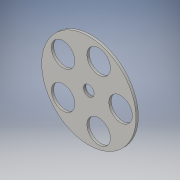
# Autodesk Inventor part: Drehplatte_Rahmenvorrrichtung
Saved by Autodesk Inventor 2016 (Build 200138000, 138)
## iProperties
Created: 2017-09-29
Part Number: Drehplatte_Rahmenvorrrichtung
Material: Generisch
Document SubType Name: Modeling
Designer: Dominik
Density: 1 g/cm^3
Appearance: Vorgabe
Author: Dominik
Autodesk Inventor part; units mm, degrees
ref_plane "YZ Plane" through (0, 0, 0) normal (1, 0, 0) x (0, 1, 0)
ref_plane "XZ Plane" through (0, 0, 0) normal (0, 1, 0) x (-1, 0, 0)
ref_plane "XY Plane" through (0, 0, 0) normal (0, 0, 1) x (1, 0, 0)
sketch "Skizze1" plane through (0, 0, 0) normal (0, 1, 0) x (-1, 0, 0)
  circle A0 centre (0, 0) radius 200
  dimension "d0" = 400
  constraints: 1 centre point, 1 coincident
  measures "d0" diameter of A0
extrude "Extrusion1" add sketch "Skizze1" along normal blind 10
sketch "Skizze2" plane through (0, 10, 0) normal (0, 1, 0) x (1, 0, 0)
  circle A0 centre (0, 0) radius 200 projected
  line L0 (0, 0) -> (200, 0) construction
  line L1 (0, 0) -> (61.8034, 190.2113)
  line L2 (0, 0) -> (200, 0) construction
  line L3 (0, 0) -> (-161.8034, 117.5571)
  line L4 (0, 0) -> (200, 0) construction
  line L5 (0, 0) -> (61.8034, -190.2113)
  line L6 (0, 0) -> (-161.8034, -117.5571)
  line L7 (0, 0) -> (200, 0)
  line L8 (200, 0) -> (100, 0)
  line L9 (0, 0) -> (30.9017, -95.1057)
  line L10 (200, 0) -> (135, 0)
  circle A1 centre (135, 0) radius 50
  line L11 (61.8034, -190.2113) -> (41.7173, -128.3926)
  circle A2 centre (41.7173, -128.3926) radius 50
  line L12 (-161.8034, -117.5571) -> (-109.2173, -79.351)
  circle A3 centre (-109.2173, -79.351) radius 50
  line L13 (-161.8034, 117.5571) -> (-109.2173, 79.351)
  circle A4 centre (-109.2173, 79.351) radius 50
  line L14 (61.8034, 190.2113) -> (41.7173, 128.3926)
  circle A5 centre (41.7173, 128.3926) radius 50
  dimension "d4" = 72
  dimension "d5" = 144
  dimension "d9" = 65
  dimension "d10" = 100
  dimension "d11" = 65
  dimension "d12" = 100
  dimension "d13" = 65
  dimension "d14" = 100
  dimension "d15" = 65
  dimension "d16" = 100
  dimension "d17" = 65
  dimension "d18" = 100
  constraints: 30 end point, 6 point on line, 5 centre point, 5 point on circle, 4 coincident, 4 horizontal, 2 equal length, 2 midpoint
  measures "d4" angle of L2 L1
  measures "d5" angle of L4 L3
  measures "d9" distance of L4.end L10.end
  measures "d10" diameter of A1
  measures "d11" distance of L11.start L11.end
  measures "d12" diameter of A2
  measures "d13" distance of L6.end L12.end
  measures "d14" diameter of A3
  measures "d15" distance of L3.end L13.end
  measures "d16" diameter of A4
  measures "d17" distance of L1.end L14.end
  measures "d18" diameter of A5
extrude "Extrusion4" cut sketch "Skizze2" against normal blind 10 contours A1 L7 | L7 A1 | A5 L1 | L1 A5 | A2 L5 | L5 A2 | A4 L3 | L3 A4 | A3 L6 | L6 A3
sketch "Skizze5" plane through (0, 0, 0) normal (0, -1, 0) x (1, 0, 0)
  circle A0 centre (0, 0) radius 22.5
  dimension "d27" = 45
  constraints: 1 centre point, 1 coincident
  measures "d27" diameter of A0
extrude "Extrusion5" cut sketch "Skizze5" against normal blind 10
